Differential Drive Robot (Autodesk Fusion 360 design; units mm, degrees)
Autodesk Fusion 360 part; units mm, degrees
ref_plane "WorkPlane1" through (0, 0, 40) normal (0, 0, 1) x (1, 0, 0) in component "base_link"
sketch "Chassis enclosure profile" plane through (0, 0, 40) normal (0, 0, 1) x (1, 0, 0) in component "base_link"
  line L0 (240, 120) -> (-60, 120)
  line L1 (-60, 120) -> (-60, -120)
  line L2 (-60, -120) -> (240, -120)
  line L3 (240, -120) -> (240, 120)
  dimension "d18" = 300
  dimension "d19" = 240
  measures "d18" horizontal distance of L0.start L0.end
  measures "d19" vertical distance of L0.end L1.end
extrude "Chassis enclosure" add sketch "Chassis enclosure profile" along normal mid plane 100 makes body 1 in component "base_link"
ref_plane "WorkPlane2" through (0, 0, 40) normal (0, 0, 1) x (1, 0, 0) in component "base_link"
sketch "Hollow interior profile" plane through (0, 0, 40) normal (0, 0, 1) x (1, 0, 0) in component "base_link"
  line L0 (237, 117) -> (-57, 117)
  line L1 (-57, 117) -> (-57, -117)
  line L2 (-57, -117) -> (237, -117)
  line L3 (237, -117) -> (237, 117)
  dimension "d24" = 294
  dimension "d25" = 234
  measures "d24" horizontal distance of L0.start L0.end
  measures "d25" vertical distance of L0.end L1.end
extrude "Hollow interior" cut sketch "Hollow interior profile" along normal mid plane 94 bodies 1 in component "base_link"
ref_plane "WorkPlane1" through (0, 0, 0) normal (0, 1, 0) x (0, 0, 1) in component "left_wheel_link"
sketch "Rubber wheel profile" plane through (0, 0, 0) normal (0, 1, 0) x (1, 0, 0) in component "left_wheel_link"
  circle A0 centre (0, 0) radius 75
  dimension "d30" = 150
  measures "d30" diameter of A0
extrude "Rubber wheel" add sketch "Rubber wheel profile" along normal mid plane 30 separate body makes body 2 in component "left_wheel_link"
ref_plane "WorkPlane2" through (0, 15.5, 0) normal (0, 1, 0) x (0, 0, 1) in component "left_wheel_link"
sketch "Outer hub profile" plane through (0, 15.5, 0) normal (0, 1, 0) x (1, 0, 0) in component "left_wheel_link"
  circle A0 centre (0, 0) radius 42.5
  dimension "d35" = 85
  measures "d35" diameter of A0
extrude "Outer hub" add sketch "Outer hub profile" along normal mid plane 1 separate body makes body 3 in component "left_wheel_link"
ref_plane "WorkPlane3" through (0, 16.5, 0) normal (0, 1, 0) x (0, 0, 1) in component "left_wheel_link"
sketch "Axle cap profile" plane through (0, 16.5, 0) normal (0, 1, 0) x (1, 0, 0) in component "left_wheel_link"
  circle A0 centre (0, 0) radius 11
  dimension "d40" = 22
  measures "d40" diameter of A0
extrude "Axle cap" add sketch "Axle cap profile" along normal mid plane 2 separate body makes body 4 in component "left_wheel_link"
ref_plane "WorkPlane1" through (0, 0, 0) normal (0, 1, 0) x (0, 0, 1) in component "right_wheel_link"
sketch "Rubber wheel profile (2)" plane through (0, 0, 0) normal (0, 1, 0) x (1, 0, 0) in component "right_wheel_link"
  circle A0 centre (0, 0) radius 75
  dimension "d45" = 150
  measures "d45" diameter of A0
extrude "Rubber wheel'" add sketch "Rubber wheel profile (2)" along normal mid plane 30 separate body makes body 5 in component "right_wheel_link"
ref_plane "WorkPlane2" through (0, -15.5, 0) normal (0, 1, 0) x (0, 0, 1) in component "right_wheel_link"
sketch "Outer hub profile (2)" plane through (0, -15.5, 0) normal (0, 1, 0) x (1, 0, 0) in component "right_wheel_link"
  circle A0 centre (0, 0) radius 42.5
  dimension "d50" = 85
  measures "d50" diameter of A0
extrude "Outer hub'" add sketch "Outer hub profile (2)" along normal mid plane 1 separate body makes body 6 in component "right_wheel_link"
ref_plane "WorkPlane3" through (0, -16.5, 0) normal (0, 1, 0) x (0, 0, 1) in component "right_wheel_link"
sketch "Axle cap profile (2)" plane through (0, -16.5, 0) normal (0, 1, 0) x (1, 0, 0) in component "right_wheel_link"
  circle A0 centre (0, 0) radius 11
  dimension "d55" = 22
  measures "d55" diameter of A0
extrude "Axle cap'" add sketch "Axle cap profile (2)" along normal mid plane 2 separate body makes body 7 in component "right_wheel_link"
ref_plane "WorkPlane1" through (0, 0, -1.5) normal (0, 0, 1) x (1, 0, 0) in component "caster_fork_link"
sketch "Swivel plate profile" plane through (0, 0, -1.5) normal (0, 0, 1) x (1, 0, 0) in component "caster_fork_link"
  circle A0 centre (0, 0) radius 22
  dimension "d60" = 44
  measures "d60" diameter of A0
extrude "Swivel plate" add sketch "Swivel plate profile" along normal mid plane 3 separate body makes body 8 in component "caster_fork_link"
ref_plane "WorkPlane2" through (0, 0, -22) normal (0, 0, 1) x (1, 0, 0) in component "caster_fork_link"
sketch "Fork left profile" plane through (0, 0, -22) normal (0, 0, 1) x (1, 0, 0) in component "caster_fork_link"
  line L0 (5, 14) -> (-20, 14)
  line L1 (-20, 14) -> (-20, 10)
  line L2 (-20, 10) -> (5, 10)
  line L3 (5, 10) -> (5, 14)
  dimension "d65" = 25
  dimension "d66" = 4
  measures "d65" horizontal distance of L0.start L0.end
  measures "d66" vertical distance of L0.end L1.end
extrude "Fork left" add sketch "Fork left profile" along normal mid plane 38 separate body makes body 9 in component "caster_fork_link"
ref_plane "WorkPlane3" through (0, 0, -22) normal (0, 0, 1) x (1, 0, 0) in component "caster_fork_link"
sketch "Fork right profile" plane through (0, 0, -22) normal (0, 0, 1) x (1, 0, 0) in component "caster_fork_link"
  line L0 (5, -10) -> (-20, -10)
  line L1 (-20, -10) -> (-20, -14)
  line L2 (-20, -14) -> (5, -14)
  line L3 (5, -14) -> (5, -10)
  dimension "d71" = 25
  dimension "d72" = 4
  measures "d71" horizontal distance of L0.start L0.end
  measures "d72" vertical distance of L0.end L1.end
extrude "Fork right" add sketch "Fork right profile" along normal mid plane 38 separate body makes body 10 in component "caster_fork_link"
ref_plane "WorkPlane1" through (0, 0, 0) normal (0, 1, 0) x (0, 0, 1) in component "caster_wheel_link"
sketch "Caster tyre profile" plane through (0, 0, 0) normal (0, 1, 0) x (1, 0, 0) in component "caster_wheel_link"
  circle A0 centre (0, 0) radius 25
  dimension "d77" = 50
  measures "d77" diameter of A0
extrude "Caster tyre" add sketch "Caster tyre profile" along normal mid plane 18 separate body makes body 11 in component "caster_wheel_link"
ref_plane "WorkPlane2" through (0, 0, 0) normal (0, 1, 0) x (0, 0, 1) in component "caster_wheel_link"
sketch "Caster axle profile" plane through (0, 0, 0) normal (0, 1, 0) x (1, 0, 0) in component "caster_wheel_link"
  circle A0 centre (0, 0) radius 5
  dimension "d82" = 10
  measures "d82" diameter of A0
extrude "Caster axle" add sketch "Caster axle profile" along normal mid plane 30 separate body makes body 12 in component "caster_wheel_link"
ref_plane "WorkPlane1" through (0, 0, -39) normal (0, 0, 1) x (1, 0, 0) in component "lidar_link"
sketch "LiDAR mount profile" plane through (0, 0, -39) normal (0, 0, 1) x (1, 0, 0) in component "lidar_link"
  line L0 (45, 45) -> (-45, 45)
  line L1 (-45, 45) -> (-45, -45)
  line L2 (-45, -45) -> (45, -45)
  line L3 (45, -45) -> (45, 45)
  dimension "d87" = 90
  dimension "d88" = 90
  measures "d87" horizontal distance of L0.start L0.end
  measures "d88" vertical distance of L0.end L1.end
extrude "LiDAR mount" add sketch "LiDAR mount profile" along normal mid plane 3 separate body makes body 13 in component "lidar_link"
ref_plane "WorkPlane2" through (0, 0, -25) normal (0, 0, 1) x (1, 0, 0) in component "lidar_link"
sketch "LiDAR lower housing profile" plane through (0, 0, -25) normal (0, 0, 1) x (1, 0, 0) in component "lidar_link"
  circle A0 centre (0, 0) radius 40
  dimension "d93" = 80
  measures "d93" diameter of A0
extrude "LiDAR lower housing" add sketch "LiDAR lower housing profile" along normal mid plane 25 separate body makes body 14 in component "lidar_link"
ref_plane "WorkPlane3" through (0, 0, 0) normal (0, 0, 1) x (1, 0, 0) in component "lidar_link"
sketch "LiDAR optical window profile" plane through (0, 0, 0) normal (0, 0, 1) x (1, 0, 0) in component "lidar_link"
  circle A0 centre (0, 0) radius 40
  dimension "d98" = 80
  measures "d98" diameter of A0
extrude "LiDAR optical window" add sketch "LiDAR optical window profile" along normal mid plane 25 separate body makes body 15 in component "lidar_link"
ref_plane "WorkPlane4" through (0, 0, 17.5) normal (0, 0, 1) x (1, 0, 0) in component "lidar_link"
sketch "LiDAR cap profile" plane through (0, 0, 17.5) normal (0, 0, 1) x (1, 0, 0) in component "lidar_link"
  circle A0 centre (0, 0) radius 40
  dimension "d103" = 80
  measures "d103" diameter of A0
extrude "LiDAR cap" add sketch "LiDAR cap profile" along normal mid plane 10 separate body makes body 16 in component "lidar_link"
ref_plane "WorkPlane1" through (0, 0, 75) normal (0, 0, 1) x (1, 0, 0)
sketch "left_wheel_joint datum" plane through (0, 0, 75) normal (0, 0, 1) x (1, 0, 0)
  point P0 (0, 145)
ref_plane "WorkPlane2" through (0, 0, 75) normal (0, 0, 1) x (1, 0, 0)
sketch "right_wheel_joint datum" plane through (0, 0, 75) normal (0, 0, 1) x (1, 0, 0)
  point P0 (0, -145)
ref_plane "WorkPlane3" through (0, 0, 65) normal (0, 0, 1) x (1, 0, 0)
sketch "caster_swivel_joint datum" plane through (0, 0, 65) normal (0, 0, 1) x (1, 0, 0)
  point P0 (200, 0)
ref_plane "WorkPlane4" through (0, 0, 25) normal (0, 0, 1) x (1, 0, 0)
sketch "caster_wheel_joint datum" plane through (0, 0, 25) normal (0, 0, 1) x (1, 0, 0)
  point P0 (185, 0)
component "base_link" placed x (1, 0, 0) y (0, 1, 0) z (0, 0, 1) at (0, 0, 75)
component "left_wheel_link" placed x (1, 0, 0) y (0, 1, 0) z (0, 0, 1) at (0, 145, 75)
component "right_wheel_link" placed x (1, 0, 0) y (0, 1, 0) z (0, 0, 1) at (0, -145, 75)
component "caster_fork_link" placed x (1, 0, 0) y (0, 1, 0) z (0, 0, 1) at (200, 0, 65)
component "caster_wheel_link" placed x (1, 0, 0) y (0, 1, 0) z (0, 0, 1) at (185, 0, 25)
component "lidar_link" placed x (1, 0, 0) y (0, 1, 0) z (0, 0, 1) at (90, 0, 205.5)
component "Differential Drive Robot v1" placed x (1, 0, 0) y (0, 1, 0) z (0, 0, 1) at (0, 0, 0) in component "caster_fork_link"
equation "chassis_length = 300 mm" comment "Differential drive robot principal dimension"
equation "chassis_width = 240 mm" comment "Differential drive robot principal dimension"
equation "chassis_height = 100 mm" comment "Differential drive robot principal dimension"
equation "panel_thickness = 3 mm" comment "Differential drive robot principal dimension"
equation "wheel_diameter = 150 mm" comment "Differential drive robot principal dimension"
equation "wheel_width = 30 mm" comment "Differential drive robot principal dimension"
equation "wheel_separation = 290 mm" comment "Differential drive robot principal dimension"
equation "ground_clearance = 65 mm" comment "Differential drive robot principal dimension"
equation "axle_offset = 90 mm" comment "Differential drive robot principal dimension"
equation "caster_diameter = 50 mm" comment "Differential drive robot principal dimension"
equation "caster_width = 18 mm" comment "Differential drive robot principal dimension"
equation "caster_pivot_x = 200 mm" comment "Differential drive robot principal dimension"
equation "caster_trail = 15 mm" comment "Differential drive robot principal dimension"
equation "lidar_diameter = 80 mm" comment "Differential drive robot principal dimension"
equation "lidar_height = 60 mm" comment "Differential drive robot principal dimension"
equation "d16 = ground_clearance + chassis_height / 2 - wheel_diameter / 2"
equation "d18 = chassis_length"
equation "d19 = chassis_width"
equation "d20 = chassis_height"
equation "d22 = ground_clearance + chassis_height / 2 - wheel_diameter / 2"
equation "d24 = chassis_length - 2 * panel_thickness"
equation "d25 = chassis_width - 2 * panel_thickness"
equation "d26 = chassis_height - 2 * panel_thickness"
equation "d30 = wheel_diameter"
equation "d31 = wheel_width"
equation "d33 = ( wheel_width / 2 + 0.5 mm )"
equation "d38 = ( wheel_width / 2 + 1.5 mm )"
equation "d45 = wheel_diameter"
equation "d46 = wheel_width"
equation "d48 = -( wheel_width / 2 + 0.5 mm )"
equation "d53 = -( wheel_width / 2 + 1.5 mm )"
equation "d77 = caster_diameter"
equation "d78 = caster_width"
equation "d85 = ( -1.5 mm ) - 37.5 mm"
equation "d91 = ( 12.5 mm ) - 37.5 mm"
equation "d93 = lidar_diameter"
equation "d96 = ( 37.5 mm ) - 37.5 mm"
equation "d98 = lidar_diameter"
equation "d101 = ( lidar_height - 5 mm ) - 37.5 mm"
equation "d103 = lidar_diameter"
named bodies: "Chassis enclosure", "Rubber wheel", "Outer hub", "Axle cap", "Swivel plate", "Fork left", "Fork right", "Caster tyre", "Caster axle", "LiDAR mount", "LiDAR lower housing", "LiDAR optical window", "LiDAR cap"
